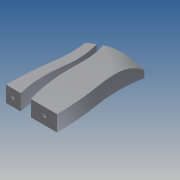
# Autodesk Inventor part: UA-70 Denkmal1
Saved by Autodesk Inventor 2014 SP2 (Build 180246200, 246)
## iProperties
Created: 2014-07-02
Part Number: UA-70 Denkmal1
Material: Allgemein
Document SubType Name: Modeling
Designer: Semenov
Density: 1 g/cm^3
Appearance: Vorgabe
Author: Semenov
Autodesk Inventor part; units mm, degrees
ref_plane "YZ Plane" through (0, 0, 0) normal (1, 0, 0) x (0, 1, 0)
ref_plane "XY Plane" through (0, 0, 0) normal (0, 0, 1) x (1, 0, 0)
sketch "Skizze3" plane through (0, 0, 0) normal (0, 0, 1) x (1, 0, 0)
  line L0 (-225, 400) -> (225, 400)
  line L1 (225, 400) -> (225, -400)
  line L2 (225, -400) -> (-225, -400)
  line L3 (-225, -400) -> (-225, 400)
  arc A0 (-195.1149, 0) -> (-225, -400) centre (2466.8593, -400) ccw
  arc A1 (-195.1149, 0) -> (-195, 270) centre (-1096.0822, 135.3833) ccw
  arc A2 (225, -400) -> (191.0498, 0) centre (-2148.3658, -400) ccw
  arc A3 (195, 400) -> (191.0498, 0) centre (1296.9948, 189.0977) ccw
  arc A4 (195, 400) -> (-98.428, 330) centre (195, -250) ccw
  arc A5 (-112.8051, 0) -> (-95, -400) centre (880.9564, -156.1612) ccw
  arc A6 (-112.8051, 0) -> (-145, 340) centre (-793.9104, 107.0299) ccw
  arc A7 (-135, 310) -> (-195, 270) centre (195, -250) ccw
  arc A8 (-65, 0) -> (-5, -400) centre (1298.3333, 0) ccw
  arc A9 (-98.428, 330) -> (-135, 310) centre (195, -250) ccw construction
  line L4 (-65, 0) -> (-65, 238.5671) construction
  arc A10 (-65, 142.5015) -> (-115, 370) centre (-607.5556, 142.5015) ccw
  line L5 (-65, 142.5015) -> (-65, 0)
  arc A11 (-115, 370) -> (-145, 340) centre (-60.8986, 285.8986) ccw
  arc A12 (-98.428, 330) -> (-225, 400) centre (-144761.9711, -261097.0223) ccw
  arc A13 (175.6814, 150) -> (-98.428, 330) centre (-1149.0878, -1568.6875) ccw
  point P0 (0, 0)
  point P1 (-225.0722, 0)
  point P2 (0, 400.05)
  point P3 (-225, 0)
  point P4 (0, 400)
  dimension "d5" = 800
  dimension "d8" = 450
  dimension "d9" = 670
  dimension "d10" = 30
  dimension "d11" = 40
  dimension "d12" = 30
  dimension "d14" = 50
  dimension "d16" = 130
  dimension "d18" = 90
  dimension "d19" = 740
  dimension "d21" = 90
  dimension "d22" = 230
  dimension "d23" = 140
  dimension "d26" = 100
  dimension "d28" = 730
  dimension "d34" = 160
  dimension "d35" = 30
  dimension "d36" = 770
  dimension "d38" = 100
  dimension "d51" = 323.428
  dimension "d52" = 250
  dimension "d53" = 2170
  constraints: 32 point on circle, 14 centre point, 12 end point, 12 tangent, 6 horizontal alignment, 4 point on line, 3 parallel, 2 midpoint, 2 vertical alignment, 1 collinear, 1 horizontal, 1 perpendicular
  measures "d5" distance of L2.end L0.start
  measures "d8" distance of L0.start L0.end
  measures "d9" distance from line of A1.end L2
  measures "d10" distance from line of A1.end L3
  measures "d11" distance edge to line of A1 L3
  measures "d12" distance from line of A3.start L1
  measures "d14" distance edge to line of A3 L1
  measures "d16" distance from line of A5.end L3
  measures "d18" distance from line of A7.start L3
  measures "d19" distance from line of A6.end L2
  measures "d21" distance of A8.end A5.end
  measures "d22" distance from line of L1 A8.end
  measures "d23" horizontal distance of A8.end A6.end
  measures "d26" distance edge to line of A5 L3
  measures "d28" distance from line of A4.end L2
  measures "d34" distance between parallel lines of L4 L3
  measures "d35" horizontal distance of A10.end A6.end
  measures "d36" distance from line of L2 A10.end
  measures "d38" radius of A11
  measures "d51" distance from line of A4.end L1
  measures "d52" distance from line of A13.start L0
  measures "d53" radius of A13
extrude "Extrusion2" add sketch "Skizze3" against normal blind 140 contours A3 A13 A4 | A0 A1 A7 A6 A5 L2 | A3 A2 L2 A8 L5 A10 A13
ref_plane "Arbeitsebene4" through (175.6814, 150, 0) normal (0, 1, 0) x (-1, 0, 0)
sketch "Skizze7" plane through (175.6814, 150, 0) normal (0, 1, 0) x (-1, 0, 0)
  line L0 (0, 0) -> (-450, 0) construction
  line L1 (-450, 0) -> (-450, -90) construction
  line L2 (-450, -90) -> (0, -90) construction
  line L3 (0, -90) -> (0, 0) construction
  arc A0 (0, 0) -> (-450, -90) centre (0, -1170) ccw
  line L4 (-450, -90) -> (-500, 50)
  line L5 (-500, 50) -> (0, 50)
  line L6 (0, 50) -> (0, 0)
  point P0 (175.6814, 0)
  dimension "d54" = 450
  dimension "d55" = 90
  dimension "d56" = 50
  dimension "d57" = 50
  constraints: 14 end point, 2 parallel, 2 perpendicular, 2 point on circle, 1 centre point, 1 collinear, 1 horizontal, 1 tangent
  measures "d54" distance of L0.start L0.end
  measures "d55" distance of L0.end L1.end
  measures "d56" distance of L5.end L0.start
  measures "d57" distance from line of L4.end L1
sweep "Sweeping1" cut profiles "Skizze7" path "Skizze3" keep normal constant yes path curves A13 A12
sketch "Skizze8" plane through (-225, -400, 0) normal (0, -1, 0) x (1, 0, 0)
  line L0 (0, 0) -> (0, -140) projected
  line L1 (130, -140) -> (0, -140) projected
  circle A0 centre (60, -70) radius 12.5
  circle A1 centre (340, -70) radius 12.5
  line L2 (450, 0) -> (450, -140) projected
  point P0 (225, 0)
  dimension "d59" = 25
  dimension "d60" = 70
  dimension "d61" = 60
  dimension "d62" = 110
  constraints: 2 centre point, 1 equal radius, 1 horizontal alignment
  measures "d59" diameter of A0
  measures "d60" distance from line of A0.centre L1
  measures "d61" distance from line of A0.centre L0
  measures "d62" distance from line of A1.centre L2
extrude "Extrusion3" cut sketch "Skizze8" against normal blind 100
equation "\"d57\" = d56"
